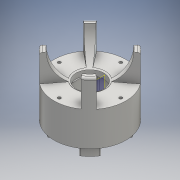
# Autodesk Inventor part: left_orbit
Saved by Autodesk Inventor 2016 (Build 200138000, 138)
## iProperties
Created: 2016-03-27
Part Number: left_orbit
Material: ABS Plastic
Document SubType Name: Modeling
Designer: Hamid Osooli
Density: 1.06 g/cm^3
Appearance: Smooth - White
Mass: 117.411 g
Surface Area: 246.095 cm^2
Volume: 110.765 cm^3
GlobalPropertyList: <PropertyList/>
Author: Hamid Osooli
Autodesk Inventor part; units mm, degrees
ref_plane "YZ Plane" through (0, 0, 0) normal (1, 0, 0) x (0, 1, 0)
ref_plane "XZ Plane" through (0, 0, 0) normal (0, 1, 0) x (-1, 0, 0)
ref_plane "XY Plane" through (0, 0, 0) normal (0, 0, 1) x (1, 0, 0)
sketch "Sketch1" plane through (0, 0, 0) normal (0, 0, 1) x (1, 0, 0)
  circle A0 centre (0, 0) radius 35
  dimension "d0" = 70
  constraints: 1 centre point, 1 coincident
  measures "d0" diameter of A0
extrude "Extrusion1" add sketch "Sketch1" against normal blind 60
sketch "Sketch16" plane through (0, 0, 0) normal (0, 0, 1) x (1, 0, 0)
  line L0 (0, 30.5) -> (0, -30.5)
  arc A0 (0, -30.5) -> (0, 30.5) centre (0, 0) ccw
  point P0 (0, 0)
  dimension "d72" = 61
  dimension "d73" = 30.5
  constraints: 2 end point, 2 point on circle, 1 centre point, 1 vertical
  measures "d72" distance of L0.start L0.end
  measures "d73" radius of A0
fillet "Fillet8" radius 2 1 edges at (-35, 0, 0)
ref_plane "Work Plane7" through (0, 0, -60) normal (0, 0, -1) x (-1, 0, 0)
sketch "Sketch42" plane through (0, 0, -60) normal (0, 0, -1) x (-1, 0, 0)
  circle A0 centre (0, 30) radius 1.5
  point P0 (0, 0)
  dimension "d468" = 3
  constraints: 1 centre point
  measures "d468" diameter of A0
ref_plane "Work Plane6" through (0, 0, -60) normal (0, 0, -1) x (-1, 0, 0)
sketch "Sketch43" plane through (0, 0, -60) normal (0, 0, -1) x (-1, 0, 0)
  circle A0 centre (30, 0) radius 1.5
  point P0 (0, 0)
  dimension "d465" = 3
  constraints: 1 centre point
  measures "d465" diameter of A0
ref_plane "Work Plane5" through (0, 0, -60) normal (0, 0, -1) x (-1, 0, 0)
sketch "Sketch44" plane through (0, 0, -60) normal (0, 0, -1) x (-1, 0, 0)
  circle A0 centre (-30, 0) radius 1.5
  point P0 (0, 0)
  dimension "d466" = 3
  constraints: 1 centre point
  measures "d466" diameter of A0
ref_plane "Work Plane4" through (0, 0, -60) normal (0, 0, -1) x (-1, 0, 0)
sketch "Sketch45" plane through (0, 0, -60) normal (0, 0, -1) x (-1, 0, 0)
  circle A0 centre (0, -30) radius 1.5
  point P0 (0, 0)
  dimension "d467" = 3
  constraints: 1 centre point
  measures "d467" diameter of A0
ref_plane "Work Plane3" through (0, 0, -60) normal (0, 0, -1) x (-1, 0, 0)
sketch "Sketch47" plane through (0, 0, -60) normal (0, 0, -1) x (-1, 0, 0)
  line L0 (8.6641, 18.25) -> (-8.6641, 18.25)
  line L1 (-12.25, 13.8079) -> (-12.25, -13.8079)
  line L2 (-8.6641, -18.25) -> (8.6641, -18.25)
  line L3 (12.25, -13.8079) -> (12.25, 13.8079)
  line L4 (-10.3414, 17.3393) -> (-11.9273, 14.8972)
  line L5 (10.3414, 17.3393) -> (11.9273, 14.8972)
  line L6 (-10.3414, -17.3393) -> (-11.9273, -14.8972)
  line L7 (10.3414, -17.3393) -> (11.9273, -14.8972)
  arc A0 (-8.6641, 18.25) -> (-10.3414, 17.3393) centre (-8.6641, 16.25) ccw
  arc A1 (-11.9273, 14.8972) -> (-12.25, 13.8079) centre (-10.25, 13.8079) ccw
  arc A2 (10.3414, 17.3393) -> (8.6641, 18.25) centre (8.6641, 16.25) ccw
  arc A3 (12.25, 13.8079) -> (11.9273, 14.8972) centre (10.25, 13.8079) ccw
  arc A4 (11.9273, -14.8972) -> (12.25, -13.8079) centre (10.25, -13.8079) ccw
  arc A5 (8.6641, -18.25) -> (10.3414, -17.3393) centre (8.6641, -16.25) ccw
  arc A6 (-10.3414, -17.3393) -> (-8.6641, -18.25) centre (-8.6641, -16.25) ccw
  arc A7 (-12.25, -13.8079) -> (-11.9273, -14.8972) centre (-10.25, -13.8079) ccw
  point P0 (12.25, 18.25)
  point P1 (-12.25, -18.25)
  point P2 (-12.25, 18.25)
  point P3 (12.25, -18.25)
  point P4 (-9.75, 18.25)
  point P5 (9.75, 18.25)
  point P6 (-9.75, -18.25)
  point P7 (9.75, -18.25)
  dimension "d417" = 24.5
  dimension "d418" = 36.5
  dimension "d419" = 2.5
  dimension "d420" = 57
  dimension "d421" = 2.5
  dimension "d422" = 57
  dimension "d423" = 2.5
  dimension "d424" = 57
  dimension "d425" = 2.5
  dimension "d426" = 57
  dimension "d427" = 2
  constraints: 16 end point, 16 point on circle, 16 point on line, 16 tangent, 8 centre point, 7 equal radius, 2 parallel, 1 horizontal, 1 perpendicular
  measures "d417" distance of point (12.25, -18.25) point (-12.25, -18.25)
  measures "d418" distance of point (-12.25, -18.25) point (-12.25, 18.25)
  measures "d419" distance of point (-9.75, 18.25) point (-12.25, 18.25)
  measures "d420" angle of L0 L4
  measures "d421" distance of point (9.75, 18.25) point (12.25, 18.25)
  measures "d422" angle of L0 L5
  measures "d423" distance of point (-9.75, -18.25) point (-12.25, -18.25)
  measures "d424" angle of L2 L6
  measures "d425" distance of point (9.75, -18.25) point (12.25, -18.25)
  measures "d426" angle of L2 L7
  measures "d427" radius of A0
extrude "Extrusion11" cut sketch "Sketch47" against normal blind 27.5
sketch "Sketch49" plane through (0, 0, -60) normal (0, 0, -1) x (-1, 0, 0)
  line L0 (0, 0) -> (30, 0) construction
  line L1 (0, 0) -> (30, 0) construction
  arc A0 (25.8489, 15.2262) -> (15.2262, 25.8489) centre (0, 0) ccw
  arc A1 (21.5407, 12.6885) -> (12.6885, 21.5407) centre (0, 0) ccw
  line L2 (21.5407, 12.6885) -> (25.8489, 15.2262)
  line L3 (12.6885, 21.5407) -> (15.2262, 25.8489)
  line L4 (0, 0) -> (30, 0) construction
  line L5 (0, 0) -> (30, 0) construction
  arc A2 (-15.2262, 25.8489) -> (-25.8489, 15.2262) centre (0, 0) ccw
  arc A3 (-12.6885, 21.5407) -> (-21.5407, 12.6885) centre (0, 0) ccw
  line L6 (-25.8489, 15.2262) -> (-21.5407, 12.6885)
  line L7 (-12.6885, 21.5407) -> (-15.2262, 25.8489)
  line L8 (0, 0) -> (30, 0) construction
  line L9 (0, 0) -> (30, 0) construction
  arc A4 (15.2262, -25.8489) -> (25.8489, -15.2262) centre (0, 0) ccw
  arc A5 (12.6885, -21.5407) -> (21.5407, -12.6885) centre (0, 0) ccw
  line L10 (25.8489, -15.2262) -> (21.5407, -12.6885)
  line L11 (15.2262, -25.8489) -> (12.6885, -21.5407)
  line L12 (0, 0) -> (30, 0) construction
  line L13 (0, 0) -> (30, 0) construction
  arc A6 (-21.5407, -12.6885) -> (-12.6885, -21.5407) centre (0, 0) ccw
  arc A7 (-25.8489, -15.2262) -> (-15.2262, -25.8489) centre (0, 0) ccw
  line L14 (-25.8489, -15.2262) -> (-21.5407, -12.6885)
  line L15 (-12.6885, -21.5407) -> (-15.2262, -25.8489)
  point P0 (0, 0)
  dimension "d448" = 30
  dimension "d450" = 25
  dimension "d453" = 30
  dimension "d454" = 25
  dimension "d457" = 30
  dimension "d458" = 25
  dimension "d461" = 25
  dimension "d462" = 30
  constraints: 32 end point, 22 point on circle, 8 centre point, 8 horizontal
  measures "d448" radius of A0
  measures "d450" radius of A1
  measures "d453" radius of A2
  measures "d454" radius of A3
  measures "d457" radius of A4
  measures "d458" radius of A5
  measures "d461" radius of A6
  measures "d462" radius of A7
extrude "Extrusion12" add sketch "Sketch49" along normal blind 10
sketch "Sketch60" plane through (0, 0, -32.5) normal (0, 0, -1) x (-1, 0, 0)
  circle A0 centre (0, 0) radius 13.5
  dimension "d439" = 27
  constraints: 1 centre point
  measures "d439" diameter of A0
revolve "Revolution5" cut sketch "Sketch16" angle 180 about axis through (0, 30.5, 0) along (0, 1, 0)
ref_plane "Work Plane10" through (8, -4.5, -32.5) normal (-1, 0, 0) x (0, 0, 1)
sketch "Sketch76" plane through (0, 0, 0) normal (0, 0, 1) x (1, 0, 0)
  line L0 (0, 0) -> (35, 0) construction
  line L1 (0, 0) -> (35, 0) construction
  line L2 (0.0001, 0) -> (35, 0) construction
  line L3 (0.0001, 0) -> (35, 0) construction
  circle A0 centre (0, 0) radius 35 projected
  line L4 (0.0001, 0) -> (35, 0) construction
  line L5 (0, 0) -> (35, 0) construction
  arc A1 (27.7674, -21.3067) -> (27.7674, 21.3066) centre (0, 0) ccw
  arc A2 (11.9003, -9.1314) -> (11.9003, 9.1314) centre (0, 0) ccw
  line L6 (11.9003, 9.1314) -> (27.7674, 21.3066)
  line L7 (11.9003, -9.1314) -> (27.7674, -21.3067)
  line L8 (0, 0) -> (35.0001, 0) construction
  line L9 (0, 0) -> (35, 0) construction
  arc A3 (21.3067, 27.7673) -> (-21.3066, 27.7674) centre (0, 0) ccw
  arc A4 (9.1315, 11.9003) -> (-9.1314, 11.9003) centre (0, 0) ccw
  line L10 (9.1315, 11.9003) -> (21.3067, 27.7673)
  line L11 (-9.1314, 11.9003) -> (-21.3066, 27.7674)
  line L12 (0, 0) -> (35.0001, 0) construction
  arc A5 (-27.7674, 21.3067) -> (-27.7674, -21.3067) centre (0, 0) ccw
  arc A6 (-12.25, 8.6565) -> (-11.9003, -9.1314) centre (-0.0001, 0) ccw
  line L13 (-12.25, 8.6565) -> (-27.7674, 21.3067)
  line L14 (-11.9003, -9.1314) -> (-27.7674, -21.3067)
  line L15 (-0.0001, 0) -> (34.9999, 0) construction
  arc A7 (-21.3067, -27.7674) -> (20.0082, -28.7171) centre (0, 0) ccw
  arc A8 (-9.1314, -11.9003) -> (8.5749, -12.3073) centre (-0.0001, 0) ccw
  line L16 (-9.1314, -11.9003) -> (-21.3067, -27.7674)
  line L17 (8.5749, -12.3073) -> (20.0082, -28.7171)
  constraints: 36 end point, 25 point on circle, 10 horizontal, 8 centre point, 4 concentric
extrude "Extrusion13" cut sketch "Sketch76" against normal blind 26.7 contours A0 L7 A2 L6 | L10 A4 L11 A0 | A0 L16 A8 L17 | L13 A6 L14 A0
sketch "Sketch81" plane through (0, 0, -32.5) normal (0, 0, -1) x (-1, 0, 0)
  circle A0 centre (0.0001, -15.25) radius 1.75
  circle A1 centre (6.5001, -15.25) radius 1.75
  circle A2 centre (-6.4999, -15.25) radius 1.75
  point P0 (0, 0)
  dimension "d435" = 3.5
  dimension "d438" = 3.5
  constraints: 3 centre point
  measures "d435" diameter of A0
  measures "d438" diameter of A2
extrude "Extrusion18" add sketch "Sketch81" along normal blind 24
extrude "Extrusion19" cut sketch "Sketch60" against normal up to next
sketch "Sketch82" plane through (0, 0, -60) normal (0, 0, -1) x (-1, 0, 0)
  circle A0 centre (-14.25, -9.7407) radius 2
  point P0 (0, 0)
  dimension "d445" = 4
  constraints: 1 centre point
  measures "d445" diameter of A0
extrude "Extrusion20" cut sketch "Sketch82" against normal blind 20
fillet "Fillet18" radius 1 16 edges at (-25.8489, 15.2262, -65) (-15.2262, 25.8489, -65) (-21.5407, 12.6885, -65) (-12.6885, 21.5407, -65) (-21.5407, -12.6885, -65) (-12.6885, -21.5407, -65) (-15.2262, -25.8489, -65) (-25.8489, -15.2262, -65) (12.6885, -21.5407, -65) (15.2262, -25.8489, -65) (21.5407, -12.6885, -65) (25.8489, -15.2262, -65) (25.8489, 15.2262, -65) (15.2262, 25.8489, -65) (12.6885, 21.5407, -65) (21.5407, 12.6885, -65)
extrude "Extrusion21" cut sketch "Sketch42" against normal through all
extrude "Extrusion22" cut sketch "Sketch43" against normal through all
extrude "Extrusion23" cut sketch "Sketch45" against normal through all
extrude "Extrusion24" cut sketch "Sketch44" against normal through all
fillet "Fillet19" radius 2 2 edges at (1.5, 30, -60) (1.5, -30, -60)
equation "\"d421\" = d419"
equation "\"d422\" = d420"
equation "\"d425\" = d423"
equation "\"d426\" = d424"
body "Solid1"
